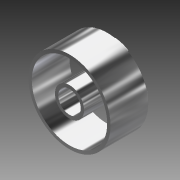
# Autodesk Inventor part: Wheety
Saved by Autodesk Inventor 2015 (Build 190159000, 159)
## iProperties
Created: 2015-01-23
Part Number: Wheety
Material: Generic
Document SubType Name: Modeling
Designer: PLTW-Stu-02
Density: 1 g/cm^3
Appearance: Chrome - Polished
Author: PLTW-Stu-02
Autodesk Inventor part; units mm, degrees
ref_plane "YZ Plane" through (0, 0, 0) normal (1, 0, 0) x (0, 1, 0)
ref_plane "XZ Plane" through (0, 0, 0) normal (0, 1, 0) x (-1, 0, 0)
sketch "Sketch1" plane through (0, 0, 0) normal (0, 0, 1) x (1, 0, 0)
  circle A0 centre (44.7782, 26.7124) radius 15.748
  circle A1 centre (44.7782, 26.7124) radius 14.478
  circle A2 centre (44.7782, 26.7124) radius 5.588
  circle A3 centre (44.7782, 26.7124) radius 4.318
  point P0 (0, 0)
  dimension "d20" = 1.27
  dimension "d21" = 8.89
  dimension "d22" = 11.176
  dimension "d23" = 1.27
  constraints: 4 centre point, 3 coincident
  measures "d20" radial gap between concentric circles of A3 A2
  measures "d21" radial gap between concentric circles of A1 A2
  measures "d22" diameter of A2
  measures "d23" radial gap between concentric circles of A0 A1
extrude "Extrusion1" add sketch "Sketch1" along normal blind 14.478
ref_plane "Work Plane1" through (44.7782, 26.7124, 0) normal (0, 0, -1) x (-1, 0, 0)
sketch "Sketch4" plane through (44.7782, 26.7124, 0) normal (0, 0, -1) x (-1, 0, 0)
  circle A0 centre (0, 0) radius 14.478 projected
  circle A1 centre (0, 0) radius 15.748 projected
  circle A2 centre (0, 0) radius 4.318 projected
  circle A3 centre (0, 0) radius 5.588 projected
  point P0 (44.7782, -26.7124)
extrude "Extrusion2" add sketch "Sketch4" along normal blind 1.27 contours A0
sketch "Sketch5" plane through (44.7782, 26.7124, -1.27) normal (0, 0, -1) x (-1, 0, 0)
  circle A0 centre (0, 0) radius 14.478 projected
  arc A1 (13.0855, 6.1954) -> (13.0855, -6.1954) centre (14.478, 0) ccw
  arc A2 (13.0855, 6.1954) -> (13.0855, -6.1954) centre (14.478, 0) ccw
  arc A3 (13.0855, -6.1954) -> (13.0855, 6.1954) centre (0, 0) ccw
  arc A4 (-1.8486, 14.3595) -> (9.9358, 10.5305) centre (4.4739, 13.7694) ccw
  arc A5 (9.9358, 10.5305) -> (-1.8486, 14.3595) centre (0, 0) ccw
  arc A6 (-14.2279, 2.6792) -> (-6.9448, 12.7036) centre (-11.7129, 8.51) ccw
  arc A7 (-6.9448, 12.7036) -> (-14.2279, 2.6792) centre (0, 0) ccw
  arc A8 (-6.9448, -12.7036) -> (-14.2279, -2.6792) centre (-11.7129, -8.51) ccw
  arc A9 (-14.2279, -2.6792) -> (-6.9448, -12.7036) centre (0, 0) ccw
  arc A10 (9.9358, -10.5305) -> (-1.8486, -14.3595) centre (4.4739, -13.7694) ccw
  arc A11 (-1.8486, -14.3595) -> (9.9358, -10.5305) centre (0, 0) ccw
  point P0 (44.7782, -26.7124)
  dimension "d16" = 360
  dimension "d24" = 6.35
  constraints: 30 point on circle, 11 centre point, 31 other
  measures "d24" radius of A1
extrude "Extrusion3" cut sketch "Sketch5" against normal through all contours A0 A1 | A4 A0 | A0 A10 | A6 A0 | A0 A8
body "Solid1"
